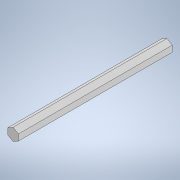
# Autodesk Inventor part: RCT-T001
Saved by Autodesk Inventor 2020 (Build 240168000, 168)
## iProperties
Created: 2019-12-05
Part Number: RCT-T001
Material: Genérico
Document SubType Name: Modeling
Designer: Frederich Schnëider
Density: 1 g/cm^3
Appearance: Valor por defecto
Author: Frederich Schnëider
Autodesk Inventor part; units mm, degrees
ref_plane "YZ Plane" through (0, 0, 0) normal (1, 0, 0) x (0, 1, 0)
ref_plane "XZ Plane" through (0, 0, 0) normal (0, 1, 0) x (-1, 0, 0)
ref_plane "XY Plane" through (0, 0, 0) normal (0, 0, 1) x (1, 0, 0)
sketch "Boceto1" plane through (0, 0, 0) normal (0, 0, 1) x (1, 0, 0)
  line L0 (-8.1086, -1.85) -> (-4.9043, -3.7)
  line L1 (-4.9043, -3.7) -> (-1.7, -1.85)
  line L2 (-1.7, -1.85) -> (-1.7, 1.85)
  line L3 (-1.7, 1.85) -> (-4.9043, 3.7)
  line L4 (-4.9043, 3.7) -> (-8.1086, 1.85)
  line L5 (-8.1086, 1.85) -> (-8.1086, -1.85)
  point P0 (0, 0)
  point P1 (0, 0)
  constraints: 12 end point, 1 vertical
extrude "Extrusión1" add sketch "Boceto1" along normal blind 92.055
